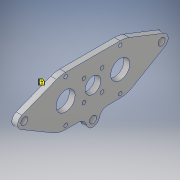
# Autodesk Inventor part: Gearbox Plate 1
Saved by Autodesk Inventor 2019.4 (Build 234330000, 330)
## iProperties
Created: 2019-12-11
Part Number: Gearbox Plate 1
Material: Aluminum 6061
Document SubType Name: Modeling
Designer: admin
Density: 2.7 g/cm^3
Appearance: Aluminum - Flat
Mass: 135.232 g
Surface Area: 199.756 cm^2
Volume: 50.0859 cm^3
Author: admin
Autodesk Inventor part; units mm, degrees
ref_plane "YZ Plane" through (0, 0, 0) normal (1, 0, 0) x (0, 1, 0)
ref_plane "XZ Plane" through (0, 0, 0) normal (0, 1, 0) x (-1, 0, 0)
ref_plane "XY Plane" through (0, 0, 0) normal (0, 0, 1) x (1, 0, 0)
sketch "Sketch1" plane through (0, 0, 0) normal (1, 0, 0) x (0, 1, 0)
  arc A0 (-30, 33.02) -> (30, 33.02) centre (0, 33.02) ccw construction
  arc A1 (30, -33.02) -> (-30, -33.02) centre (0, -33.02) ccw construction
  line L0 (0, 33.02) -> (0, -33.02) construction
  line L1 (30, 33.02) -> (30, -33.02)
  line L2 (-30, -33.02) -> (-30, 33.02)
  arc A2 (30, 33.02) -> (-30, 33.02) centre (0, 33.02) ccw
  arc A3 (-30, -33.02) -> (30, -33.02) centre (0, -33.02) ccw
  circle A4 centre (0, 0) radius 9.5
  circle A5 centre (0, 33.02) radius 11.5
  circle A6 centre (0, -33.02) radius 11.5
  dimension "d0" = 60
  dimension "d1" = 60
  dimension "d2" = 66.04
  dimension "d3" = 19
  dimension "d4" = 23
  dimension "d5" = 23
  constraints: 8 point on circle, 7 centre point, 6 end point, 4 coincident, 4 tangent, 1 midpoint, 1 vertical
  measures "d0" diameter of A0
  measures "d1" diameter of A1
  measures "d2" distance of L0.end L0.start
  measures "d3" diameter of A4
  measures "d4" diameter of A5
  measures "d5" diameter of A6
extrude "Extrusion1" add sketch "Sketch1" along normal blind 7
sketch "Sketch4" plane through (7, 0, 0) normal (1, 0, 0) x (0, 0, -1)
  circle A0 centre (33.02, 0) radius 25.4
  circle A1 centre (-33.02, 0) radius 25.4
  circle A2 centre (33.02, 0) radius 11.5 projected
  circle A3 centre (-33.02, 0) radius 11.5 projected
  circle A4 centre (33.02, 25.4) radius 2.2
  line L0 (33.02, 30) -> (-33.02, 30) projected
  circle A5 centre (11.023, 12.7) radius 2.2
  circle A6 centre (11.023, -12.7) radius 2.2
  circle A7 centre (33.02, -25.4) radius 2.2
  circle A8 centre (55.017, -12.7) radius 2.2
  circle A9 centre (55.017, 12.7) radius 2.2
  circle A10 centre (-33.02, 25.4) radius 2.2
  circle A11 centre (-55.017, 12.7) radius 2.2
  circle A12 centre (-55.017, -12.7) radius 2.2
  circle A13 centre (-33.02, -25.4) radius 2.2
  circle A14 centre (-11.023, -12.7) radius 2.2
  circle A15 centre (-11.023, 12.7) radius 2.2
  point P0 (0, 0)
  dimension "d20" = 50.8
  dimension "d21" = 50.8
  dimension "d22" = 4.4
  dimension "d23" = 4.6
  dimension "d26" = 360
  dimension "d28" = 4.4
  dimension "d29" = 4.6
  dimension "d32" = 360
  constraints: 12 centre point, 2 vertical alignment, 32 other
  measures "d22" diameter of A4
  measures "d23" distance from line of L0 A4.centre
  measures "d28" diameter of A10
  measures "d29" distance from line of L0 A10.centre
extrude "Extrusion4" cut sketch "Sketch4" against normal blind 7 contours A9 A0 | A0 A9 | A8 A0 | A0 A8 | A4 A0 | A0 A4 | A7 A0 | A0 A7 | A5 A0 | A0 A5 | A6 A0 | A0 A6 | A15 A1 | A1 A15 | A14 A1 | A1 A14 | A10 A1 | A1 A10 | A13 A1 | A1 A13 | A11 A1 | A1 A11 | A12 A1 | A1 A12
sketch "Sketch5" plane through (7, 0, 0) normal (1, 0, 0) x (0, 0, -1)
  circle A0 centre (0, -36) radius 4.25
  line L0 (-33.02, -30) -> (33.02, -30) projected
  circle A1 centre (-33.02, 0) radius 11.5 projected
  circle A2 centre (0, -36) radius 8
  arc A3 (-33.02, 30) -> (-33.02, -30) centre (-33.02, 0) ccw projected
  line L1 (0, 0) -> (0, -20)
  line L2 (0, 0) -> (20, 0) construction
  line L3 (-33.02, 30) -> (16.98, 30) construction
  arc A4 (33.02, -30) -> (33.02, 30) centre (33.02, 0) ccw projected
  arc A5 (-85.9443, 11.4464) -> (-87.0909, -2.8868) centre (-83.02, 4) ccw
  line L4 (-87.0909, -2.8868) -> (-48.286, -25.8253)
  line L5 (-85.9443, 11.4464) -> (-43.9861, 27.9239)
  line L6 (-43.9861, 27.9239) -> (-48.286, -25.8253)
  circle A6 centre (83.02, 4) radius 8
  line L7 (87.0909, -2.8868) -> (48.286, -25.8253)
  line L8 (85.9443, 11.4464) -> (43.9861, 27.9239)
  line L9 (43.9861, 27.9239) -> (48.286, -25.8253)
  dimension "d36" = 8.5
  dimension "d37" = 6
  dimension "d38" = 33.02
  dimension "d39" = 16
  dimension "d47" = 20
  dimension "d48" = 90
  dimension "d54" = 16
  dimension "d55" = 50
  dimension "d56" = 4
  constraints: 18 end point, 6 point on circle, 5 symmetric about line, 4 centre point, 4 tangent, 2 horizontal, 1 coincident, 1 perpendicular, 1 vertical, 1 other
  measures "d36" diameter of A0
  measures "d37" distance from line of L0 A0.centre
  measures "d38" horizontal distance of A1.centre A0.centre
  measures "d39" diameter of A2
  measures "d47" distance of L1.start L1.end
  measures "d48" angle of L1 L2
  measures "d54" diameter of A5
  measures "d55" horizontal distance of A1.centre A5.centre
  measures "d56" vertical distance of A1.centre A5.centre
extrude "Extrusion5" add sketch "Sketch5" against normal blind 7 contours A2 L0 | L0 A2 | L6 A3 | A3 L4 A5 L5 | L9 A4 | A4 L8 A6 L7 | A6
fillet "Fillet2" radius 10 2 edges at (3.5, -30, 5.2915) (3.5, -30, -5.2915)
sketch "Sketch6" plane through (7, 0, 0) normal (1, 0, 0) x (0, 0, -1)
  circle A0 centre (83.02, 4) radius 4.25
  arc A1 (87.0909, -2.8868) -> (85.9443, 11.4464) centre (83.02, 4) ccw projected
  circle A2 centre (-83.02, 4) radius 4.25
  arc A3 (-85.9443, 11.4464) -> (-87.0909, -2.8868) centre (-83.02, 4) ccw projected
  point P0 (0, 0)
  dimension "d51" = 8.5
  dimension "d57" = 8.5
  constraints: 2 centre point, 2 concentric
  measures "d51" diameter of A0
  measures "d57" diameter of A2
extrude "Extrusion6" cut sketch "Sketch6" against normal blind 10
body "Solid1"
